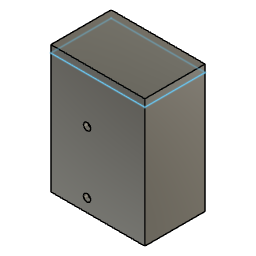
battery mount (Autodesk Fusion 360 design; units mm, degrees)
Autodesk Fusion 360 part; units mm, degrees
sketch "Sketch1" plane through (0, 0, 0) normal (0, 0, 1) x (1, 0, 0)
  line L0 (-50, 75) -> (-11, 75)
  line L1 (-11, 75) -> (-11, 50)
  line L2 (-11, 50) -> (-50, 50)
  line L3 (-50, 50) -> (-50, 75)
  line L4 (-12.8, 51.8) -> (-48.2, 51.8)
  line L5 (-48.2, 51.8) -> (-48.2, 73.2)
  line L6 (-48.2, 73.2) -> (-12.8, 73.2)
  line L7 (-12.8, 73.2) -> (-12.8, 51.8)
  dimension "d1" = 39
  dimension "d2" = 25
  dimension "d3" = 1.8
  constraint horizontal L0
  constraint vertical L1
  constraint horizontal L2
  constraint vertical L3
  measures "d1" distance of L0.start L0.end
  measures "d2" distance of L0.start L2.end
extrude "Extrude1" add sketch "Sketch1" along normal blind 50
sketch "Sketch2" plane through (0, 50, 0) normal (0, -1, 0) x (1, 0, 0)
  line L0 (-50, 0) -> (-11, 0)
  line L1 (-11, 0) -> (-11, 50)
  line L2 (-11, 50) -> (-50, 50)
  line L3 (-50, 50) -> (-50, 0)
  circle A0 centre (-35, 31) radius 1.5
  circle A1 centre (-35, 5.4) radius 1.5
  dimension "d7" = 3
  dimension "d9" = 3
  measures "d7" diameter of A0
  measures "d9" diameter of A1
extrude "Extrude2" cut sketch "Sketch2" against normal blind 11 contours A0 | A1
sketch "Sketch4" plane through (0, 0, 0) normal (0, 0, 1) x (1, 0, 0)
  line L0 (-50, 50, 50) -> (-11, 50, 50)
  line L1 (-11, 50, 50) -> (-11, 75, 50)
  line L2 (-11, 75, 50) -> (-50, 75, 50)
  line L3 (-50, 75, 50) -> (-50, 50, 50)
extrude "Extrude5" add sketch "Sketch4" along normal blind 3 contours L0 L1 L2 L3 in plane through (0, 0, 50) normal (0, 0, 1)
